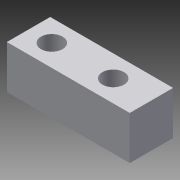
# Autodesk Inventor part: XcrRightXEndstopTrigger
Saved by Autodesk Inventor 2013 (Build 170138000, 138)
## iProperties
Created: 2015-01-14
Part Number: XcrRightXEndstopTrigger
Material: Generic
Document SubType Name: Modeling
Designer: dzban
Density: 1 g/cm^3
Author: dzban
Autodesk Inventor part; units mm, degrees
ref_plane "YZ Plane" through (0, 0, 0) normal (1, 0, 0) x (0, 1, 0)
ref_plane "XZ Plane" through (0, 0, 0) normal (0, 1, 0) x (-1, 0, 0)
ref_plane "XY Plane" through (0, 0, 0) normal (0, 0, 1) x (1, 0, 0)
sketch "Sketch1" plane through (0, 0, 0) normal (0, 0, 1) x (1, 0, 0)
  circle A0 centre (-13.7859, 3) radius 1.5
  circle A1 centre (-5.2859, 3) radius 1.5
  line L0 (0, 0) -> (-17, 0)
  line L1 (0, 6) -> (0, 0)
  line L2 (-17, 6) -> (0, 6)
  line L3 (-17, 0) -> (-17, 6)
  constraints: 8 end point, 2 centre point
extrude "Extrusion1" add sketch "Sketch1" along normal blind 6
body "Solid1"
